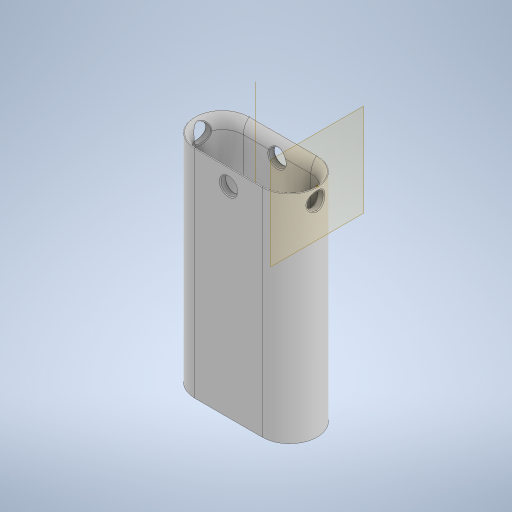
# Autodesk Inventor part: v1.0-B-battery-holder
Saved by Autodesk Inventor 2023 (Build 270158030, 158C)
## iProperties
Created: 2023-04-28
Part Number: v1.0-B-battery-holder
Material: Generic
Document SubType Name: Modeling
Designer: Imogen Heard
Density: 1 g/cm^3
Appearance: Default
Author: Imogen Heard
Autodesk Inventor part; units mm, degrees
ref_plane "YZ Plane" through (0, 0, 0) normal (1, 0, 0) x (0, 1, 0)
ref_plane "XZ Plane" through (0, 0, 0) normal (0, 1, 0) x (-1, 0, 0)
ref_plane "XY Plane" through (0, 0, 0) normal (0, 0, 1) x (1, 0, 0)
sketch "Sketch1" plane through (0, 0, 0) normal (0, 1, 0) x (-1, 0, 0)
  line L0 (8, 0) -> (-8, 0) construction
  line L1 (8, 5) -> (-8, 5)
  line L2 (-8, -5) -> (8, -5)
  arc A0 (8, -5) -> (8, 5) centre (8, 0) ccw
  arc A1 (-8, 5) -> (-8, -5) centre (-8, 0) ccw
  line L3 (8, 0) -> (-8, 0) construction
  line L4 (8, 6.5) -> (-8, 6.5)
  line L5 (-8, -6.5) -> (8, -6.5)
  arc A2 (8, -6.5) -> (8, 6.5) centre (8, 0) ccw
  arc A3 (-8, 6.5) -> (-8, -6.5) centre (-8, 0) ccw
  point P0 (0, 0)
  point P1 (0, 0)
  point P2 (-13, 0)
  point P3 (13, 0)
  point P4 (0, 0)
  dimension "d0" = 10
  dimension "d1" = 26
  dimension "d2" = 1.5
  constraints: 16 end point, 10 point on circle, 8 tangent, 4 centre point, 2 horizontal, 2 midpoint, 2 parallel, 1 coincident
  measures "d0" distance between parallel lines of L1 L2
  measures "d1" distance of point (-13, 0) point (13, 0)
  measures "d2" distance between parallel lines of L2 L5
extrude "Extrusion1" add sketch "Sketch1" along normal blind 50
sketch "Sketch2" plane through (0, 0, 0) normal (0, -1, 0) x (1, 0, 0)
  arc A0 (8, -6.5) -> (8, 6.5) centre (8, 0) ccw projected
  line L0 (-8, 6.5) -> (8, 6.5) projected
  arc A1 (-8, 6.5) -> (-8, -6.5) centre (-8, 0) ccw projected
  line L1 (8, -6.5) -> (-8, -6.5) projected
  point P0 (0, 0)
extrude "Extrusion2" add sketch "Sketch2" along normal blind 1.5
sketch "Sketch3" plane through (-8, 50, 6.5) normal (0, 0, 1) x (1, 0, 0)
  circle A0 centre (8, -4) radius 2
  line L0 (0, 0) -> (16, 0) projected
  line L1 (0, -51.5) -> (0, 0) projected
  line L2 (16, 0) -> (16, -51.5) projected
  point P0 (8, -50)
  point P1 (8, 0)
  dimension "d7" = 4
  dimension "d8" = 4
  dimension "d9" = 8
  dimension "d10" = 8
  constraints: 1 centre point, 1 midpoint
  measures "d7" diameter of A0
  measures "d8" distance of point (8, 0) A0.centre
  measures "d9" distance from line of L1 A0.centre
  measures "d10" distance from line of L2 A0.centre
extrude "Extrusion3" cut sketch "Sketch3" against normal through all
ref_plane "Work Plane1" through (14.5, 50, 0) normal (1, 0, 0) x (0, 1, 0)
sketch "Sketch4" plane through (14.5, 50, 0) normal (1, 0, 0) x (0, 1, 0)
  circle A0 centre (-3, 0) radius 2
  line L0 (0, -6.5) -> (0, 6.5) projected
  point P0 (-50, 0)
  point P1 (0, 0)
  dimension "d16" = 4
  dimension "d17" = 3
  constraints: 1 centre point, 1 horizontal alignment, 1 midpoint
  measures "d16" diameter of A0
  measures "d17" distance from line of L0 A0.centre
extrude "Extrusion4" cut sketch "Sketch4" against normal through all
fillet "Fillet1" radius 4 4 edges at (13, 50, 0) (0, 50, 5) (-13, 50, 0) (0, 50, -5)
fillet "Fillet2" radius 0.1 4 edges at (14.5, 50, 0) (0, 50, -6.5) (-14.5, 50, 0) (0, 50, 6.5)
fillet "Fillet3" radius 0.2 17 edges at (-14.4558, 45.1488, 0.757) (-2, 46, 6.5) (14.1874, 46.8162, -1.9915) (14.1847, 47.0033, 2) (-0.0001, 48, -5.1607) (1.9486, 46.4503, -5) (-0.4503, 44.0514, -5) (-2, 46, -6.5) (-0.0001, 48, 5.1607) (-0.4503, 44.0514, 5) (1.9486, 46.4503, 5) (13.0836, 48.3691, -1.4579) (13.0835, 48.369, 1.458) (13, 45, 0.001) (-13, 45, 0.001) (-13.0835, 48.369, -1.458) (-13.0836, 48.3691, 1.4579)
fillet "Fillet4" radius 3 4 edges at (0, 0, 5) (-13, 0, 0) (0, 0, -5) (13, 0, 0)
body "Solid1"
